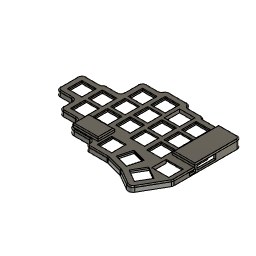
Plate (Autodesk Fusion 360 design; units mm, degrees)
Autodesk Fusion 360 part; units mm, degrees
sketch "plate-Edge_Cuts" plane through (0, 0, 0) normal (0, 0, 1) x (1, 0, 0)
  line L0 (52.0077, -29.7844) -> (52.0077, -15.8344)
  line L1 (65.9577, -29.7844) -> (52.0077, -29.7844)
  line L2 (29.9577, -38.8344) -> (29.9577, -52.7844)
  line L3 (144.4827, -45.3094) -> (142.4827, -45.3094)
  line L4 (65.9577, -49.8344) -> (65.9577, -63.7844)
  line L5 (106.0077, -65.7844) -> (106.0077, -51.8344)
  line L6 (142.4827, -45.0594) -> (144.4827, -45.0594)
  line L7 (96.4397, -85.7414) -> (100.0507, -72.2664)
  line L8 (119.9577, -48.7844) -> (106.0077, -48.7844)
  line L9 (100.0507, -72.2664) -> (113.5257, -75.8774)
  line L10 (119.9577, -34.8334) -> (119.9577, -48.7844)
  line L11 (119.9577, -51.8344) -> (119.9577, -65.7844)
  line L12 (119.9577, -65.7844) -> (106.0077, -65.7844)
  line L13 (106.0077, -34.8335) -> (119.9577, -34.8334)
  line L14 (113.5257, -75.8774) -> (109.9147, -89.3524)
  line L15 (65.9577, -63.7844) -> (52.0077, -63.7844)
  line L16 (65.9577, -15.8344) -> (65.9577, -29.7844)
  line L17 (52.0077, -49.8344) -> (65.9577, -49.8344)
  line L18 (83.9577, -25.7844) -> (70.0077, -25.7844)
  line L19 (16.0077, -52.7844) -> (16.0077, -38.8344)
  line L20 (70.0077, -25.7844) -> (70.0077, -11.8344)
  line L21 (106.0077, -48.7844) -> (106.0077, -34.8335)
  line L22 (106.0077, -51.8344) -> (119.9577, -51.8344)
  line L23 (109.9147, -89.3524) -> (96.4397, -85.7414)
  line L24 (52.0077, -63.7844) -> (52.0077, -49.8344)
  line L25 (83.9577, -11.8344) -> (83.9577, -25.7844)
  line L26 (29.9577, -52.7844) -> (16.0077, -52.7844)
  line L27 (101.9577, -63.7844) -> (88.0077, -63.7844)
  line L28 (123.4827, -78.3094) -> (123.4827, -64.3094)
  line L29 (119.9577, -17.8344) -> (119.9577, -31.7844)
  line L30 (106.0077, -31.7844) -> (106.0077, -17.8344)
  line L31 (119.9577, -31.7844) -> (106.0077, -31.7844)
  line L32 (83.9577, -28.8326) -> (83.9577, -42.7844)
  line L33 (83.9577, -59.7844) -> (70.0077, -59.7844)
  line L34 (83.9577, -42.7844) -> (70.0077, -42.7844)
  line L35 (70.0077, -42.7844) -> (70.0077, -28.8329)
  line L36 (88.0077, -49.8344) -> (101.9577, -49.8344)
  line L37 (83.9577, -45.8344) -> (83.9577, -59.7844)
  line L38 (106.0077, -17.8344) -> (119.9577, -17.8344)
  line L39 (52.0077, -15.8344) -> (65.9577, -15.8344)
  line L40 (139.9827, -78.3094) -> (123.4827, -78.3094)
  line L41 (101.9577, -49.8344) -> (101.9577, -63.7844)
  line L42 (16.0077, -38.8344) -> (29.9577, -38.8344)
  line L43 (70.0077, -11.8344) -> (83.9577, -11.8344)
  line L44 (88.0077, -63.7844) -> (88.0077, -49.8344)
  line L45 (88.0077, -15.8344) -> (101.9577, -15.8344)
  line L46 (114.4547, -91.3624) -> (121.4297, -79.2814)
  line L47 (101.9577, -32.8344) -> (101.9577, -46.7854)
  line L48 (34.0077, -36.8344) -> (47.9577, -36.8344)
  line L49 (101.9577, -46.7854) -> (88.0077, -46.7853)
  line L50 (47.9577, -53.8325) -> (47.9577, -67.7844)
  line L51 (91.4577, -71.3344) -> (91.4577, -85.2844)
  line L52 (133.5107, -86.2564) -> (126.5357, -98.3374)
  line L53 (34.0077, -53.8331) -> (47.9577, -53.8325)
  line L54 (47.9577, -67.7844) -> (34.0077, -67.7844)
  line L55 (101.9577, -15.8344) -> (101.9577, -29.7844)
  line L56 (91.4577, -85.2844) -> (77.5077, -85.2844)
  line L57 (47.9577, -36.8344) -> (47.9577, -50.7844)
  line L58 (88.0077, -29.7844) -> (88.0077, -15.8344)
  line L59 (121.4297, -79.2814) -> (133.5107, -86.2564)
  line L60 (77.5077, -71.3344) -> (91.4577, -71.3344)
  line L61 (70.0077, -45.8344) -> (83.9577, -45.8344)
  line L62 (77.5077, -85.2844) -> (77.5077, -71.3344)
  line L63 (88.0077, -46.7853) -> (88.0077, -32.8344)
  line L64 (101.9577, -29.7844) -> (88.0077, -29.7844)
  line L65 (88.0077, -32.8344) -> (101.9577, -32.8344)
  line L66 (126.5357, -98.3374) -> (114.4547, -91.3624)
  line L67 (70.0077, -59.7844) -> (70.0077, -45.8344)
  line L68 (47.9577, -50.7844) -> (34.0077, -50.7844)
  line L69 (70.0077, -28.8329) -> (83.9577, -28.8326)
  line L70 (34.0077, -67.7844) -> (34.0077, -53.8331)
  line L71 (34.0077, -50.7844) -> (34.0077, -36.8344)
  line L72 (65.9577, -46.7844) -> (52.0077, -46.7844)
  line L73 (52.0077, -46.7844) -> (52.0077, -32.8329)
  line L74 (65.9577, -32.8325) -> (65.9577, -46.7844)
  line L75 (52.0077, -32.8329) -> (65.9577, -32.8325)
  line L76 (142.4827, -57.8094) -> (144.4827, -57.8094)
  line L77 (30.4577, -38.3344) -> (30.4577, -53.2844)
  line L78 (30.4577, -53.2844) -> (15.5077, -53.2844)
  line L79 (15.5077, -53.2844) -> (15.5077, -38.3344)
  line L80 (15.5077, -38.3344) -> (30.4577, -38.3344)
  line L81 (33.5077, -36.3344) -> (48.4577, -36.3344)
  line L82 (95.8273, -86.0949) -> (99.6972, -71.654)
  line L83 (99.6972, -71.654) -> (114.1381, -75.5238)
  line L84 (114.1381, -75.5238) -> (110.2682, -89.9647)
  line L85 (110.2682, -89.9647) -> (95.8273, -86.0949)
  line L86 (105.5077, -68.2844) -> (105.5077, -51.3344)
  line L87 (105.5077, -51.3344) -> (120.4577, -51.3344)
  line L88 (120.4577, -51.3344) -> (120.4577, -68.2844)
  line L89 (120.4577, -68.2844) -> (105.5077, -68.2844)
  line L90 (105.5077, -17.3344) -> (120.4577, -17.3344)
  line L91 (87.5077, -66.2844) -> (87.5077, -32.3344)
  line L92 (87.5077, -32.3344) -> (102.4577, -32.3344)
  line L93 (102.4577, -32.3344) -> (102.4577, -66.2844)
  line L94 (69.5077, -62.7844) -> (69.5077, -45.3344)
  line L95 (69.5077, -45.3344) -> (84.4577, -45.3344)
  line L96 (84.4577, -45.3344) -> (84.4577, -62.7844)
  line L97 (84.4577, -62.7844) -> (69.5077, -62.7844)
  line L98 (69.5077, -11.3344) -> (84.4577, -11.3344)
  line L99 (66.4577, -15.3344) -> (66.4577, -47.2844)
  line L100 (66.4577, -47.2844) -> (51.5077, -47.2844)
  line L101 (51.5077, -47.2844) -> (51.5077, -15.3344)
  line L102 (48.4577, -36.3344) -> (48.4577, -68.2844)
  line L103 (48.4577, -68.2844) -> (33.5077, -68.2844)
  line L104 (33.5077, -68.2844) -> (33.5077, -36.3344)
  line L105 (66.4577, -49.3344) -> (66.4577, -64.2844)
  line L106 (66.4577, -64.2844) -> (51.5077, -64.2844)
  line L107 (51.5077, -64.2844) -> (51.5077, -49.3344)
  line L108 (51.5077, -49.3344) -> (66.4577, -49.3344)
  line L109 (51.5077, -15.3344) -> (66.4577, -15.3344)
  line L110 (69.5077, -43.2844) -> (69.5077, -11.3344)
  line L111 (84.4577, -11.3344) -> (84.4577, -43.2844)
  line L112 (84.4577, -43.2844) -> (69.5077, -43.2844)
  line L113 (102.4577, -66.2844) -> (87.5077, -66.2844)
  line L114 (87.5077, -30.2844) -> (87.5077, -15.3344)
  line L115 (87.5077, -15.3344) -> (102.4577, -15.3344)
  line L116 (102.4577, -15.3344) -> (102.4577, -30.2844)
  line L117 (102.4577, -30.2844) -> (87.5077, -30.2844)
  line L118 (105.5077, -49.2844) -> (105.5077, -17.3344)
  line L119 (120.4577, -17.3344) -> (120.4577, -49.2844)
  line L120 (120.4577, -49.2844) -> (105.5077, -49.2844)
  line L121 (77.0077, -85.7844) -> (77.0077, -68.8344)
  line L122 (77.0077, -68.8344) -> (91.9577, -68.8344)
  line L123 (91.9577, -68.8344) -> (91.9577, -85.7844)
  line L124 (91.9577, -85.7844) -> (77.0077, -85.7844)
  line L125 (113.7717, -91.5454) -> (121.2467, -78.5984)
  line L126 (121.2467, -78.5984) -> (134.1937, -86.0734)
  line L127 (134.1937, -86.0734) -> (126.7187, -99.0204)
  line L128 (126.7187, -99.0204) -> (113.7717, -91.5454)
  line L129 (51.7516, -67.7801) -> (73.7516, -67.7801)
  line L130 (73.7516, -67.7801) -> (73.7516, -80.7801)
  line L131 (73.7516, -80.7801) -> (51.7516, -80.7801)
  line L132 (51.7516, -80.7801) -> (51.7516, -67.7801)
  line L133 (75.3516, -66.1801) -> (75.3516, -82.3801)
  line L134 (75.3516, -82.3801) -> (50.1516, -82.3801)
  line L135 (50.1516, -82.3801) -> (50.1516, -66.1801)
  line L136 (50.1516, -66.1801) -> (75.3516, -66.1801)
  arc A0 (125.737, -102.2448) -> (129.1584, -101.3221) centre (126.9827, -100.0594) ccw
  arc A1 (129.1584, -101.3221) -> (129.16, -101.3193) centre (128.2935, -100.8202) ccw
  line L137 (129.16, -101.3193) -> (141.9487, -79.12)
  line L138 (142.4827, -15.8344) -> (142.4827, -77.1233)
  arc A2 (142.4827, -16.3094) -> (140.4827, -14.3094) centre (140.4827, -16.3094) ccw
  line L139 (105.4827, -14.3094) -> (140.4827, -14.3094)
  arc A3 (104.9827, -13.8094) -> (105.4827, -14.3094) centre (105.4827, -13.8094) ccw
  arc A4 (104.9827, -13.8094) -> (103.4827, -12.3094) centre (103.4827, -13.8094) ccw
  line L140 (88.4827, -12.3094) -> (103.4827, -12.3094)
  arc A5 (87.4827, -11.3094) -> (88.4827, -12.3094) centre (88.4827, -11.3094) ccw
  line L141 (87.4827, -10.3094) -> (87.4827, -11.3094)
  arc A6 (87.4827, -10.3094) -> (85.4827, -8.3094) centre (85.4827, -10.3094) ccw
  line L142 (68.4827, -8.3094) -> (85.4827, -8.3094)
  arc A7 (68.4827, -8.3094) -> (66.4827, -10.3094) centre (68.4827, -10.3094) ccw
  line L143 (66.4827, -10.3094) -> (66.4827, -11.3094)
  arc A8 (65.4827, -12.3094) -> (66.4827, -11.3094) centre (65.4827, -11.3094) ccw
  line L144 (65.4827, -12.3094) -> (50.4827, -12.3094)
  arc A9 (50.4827, -12.3094) -> (48.4827, -14.3094) centre (50.4827, -14.3094) ccw
  line L145 (48.4827, -14.3094) -> (48.4827, -32.3094)
  arc A10 (47.4827, -33.3094) -> (48.4827, -32.3094) centre (47.4827, -32.3094) ccw
  line L146 (47.4827, -33.3094) -> (32.4827, -33.3094)
  arc A11 (32.4827, -33.3094) -> (30.9827, -34.8094) centre (32.4827, -34.8094) ccw
  arc A12 (30.4827, -35.3094) -> (30.9827, -34.8094) centre (30.4827, -34.8094) ccw
  line L147 (14.4827, -35.3094) -> (30.4827, -35.3094)
  arc A13 (14.4827, -35.3094) -> (12.4827, -37.3094) centre (14.4827, -37.3094) ccw
  line L148 (12.4827, -37.3094) -> (12.4827, -54.3094)
  arc A14 (12.4827, -54.3094) -> (14.4827, -56.3094) centre (14.4827, -54.3094) ccw
  line L149 (14.4827, -56.3094) -> (29.4827, -56.3094)
  arc A15 (30.4827, -57.3094) -> (29.4827, -56.3094) centre (29.4827, -57.3094) ccw
  line L150 (30.4827, -57.3094) -> (30.4827, -69.3094)
  arc A16 (30.4827, -69.3094) -> (32.4827, -71.3094) centre (32.4827, -69.3094) ccw
  line L151 (32.4827, -71.3094) -> (50.1516, -71.3094)
  line L152 (74.9827, -88.8094) -> (92.8162, -88.8094)
  line L153 (93.995, -88.9665) -> (110.2134, -93.3687)
  line L154 (111.3021, -93.8245) -> (125.7283, -102.2398)
  arc A17 (125.7283, -102.2398) -> (125.737, -102.2448) centre (126.2322, -101.3761) ccw
  line L155 (32.4827, -73.3094) -> (44.1516, -73.3094)
  arc A18 (28.4827, -69.3094) -> (32.4827, -73.3094) centre (32.4827, -69.3094) ccw
  line L156 (28.4827, -61.3094) -> (28.4827, -69.3094)
  line L157 (14.4827, -58.3094) -> (25.4827, -58.3094)
  arc A19 (10.4827, -54.3094) -> (14.4827, -58.3094) centre (14.4827, -54.3094) ccw
  line L158 (10.4827, -37.3094) -> (10.4827, -54.3094)
  arc A20 (14.4827, -33.3094) -> (10.4827, -37.3094) centre (14.4827, -37.3094) ccw
  line L159 (14.4827, -33.3094) -> (28.7411, -33.3094)
  arc A21 (32.4827, -31.3094) -> (29.5725, -32.8649) centre (32.4827, -34.8094) ccw
  line L160 (43.4827, -31.3094) -> (32.4827, -31.3094)
  line L161 (46.4827, -14.3094) -> (46.4827, -28.3094)
  arc A22 (50.4827, -10.3094) -> (46.4827, -14.3094) centre (50.4827, -14.3094) ccw
  line L162 (62.1582, -10.3094) -> (50.4827, -10.3094)
  arc A23 (68.4827, -6.3094) -> (64.8687, -8.5951) centre (68.4827, -10.3094) ccw
  line L163 (68.4827, -6.3094) -> (85.4827, -6.3094)
  arc A24 (89.0967, -8.5951) -> (85.4827, -6.3094) centre (85.4827, -10.3094) ccw
  line L164 (91.8073, -10.3094) -> (103.4827, -10.3094)
  arc A25 (106.3929, -11.8649) -> (103.4827, -10.3094) centre (103.4827, -13.8094) ccw
  line L165 (107.2244, -12.3094) -> (140.4827, -12.3094)
  arc A26 (144.4827, -16.3094) -> (140.4827, -12.3094) centre (140.4827, -16.3094) ccw
  line L166 (144.4827, -16.3094) -> (144.4827, -77.6582)
  line L167 (130.893, -102.3177) -> (143.9487, -79.6549)
  arc A27 (130.8881, -102.3261) -> (130.893, -102.3177) centre (128.2935, -100.8202) ccw
  arc A28 (124.7466, -103.9824) -> (130.8881, -102.3261) centre (126.9827, -100.0594) ccw
  arc A29 (124.7206, -103.9674) -> (124.7466, -103.9824) centre (126.2322, -101.3761) ccw
  line L168 (110.4657, -95.6521) -> (124.7206, -103.9674)
  line L169 (93.7284, -90.9665) -> (109.498, -95.2468)
  line L170 (74.9827, -90.8094) -> (92.5496, -90.8094)
  arc A30 (48.1516, -78.3801) -> (54.1516, -84.3801) centre (54.1516, -78.3801) ccw
  line L171 (54.1516, -84.3801) -> (68.9827, -84.3801)
  line L172 (48.1516, -78.3801) -> (48.1516, -77.3094)
  arc A31 (48.1516, -77.3094) -> (44.1516, -73.3094) centre (44.1516, -77.3094) ccw
  arc A32 (71.9827, -87.3801) -> (68.9827, -84.3801) centre (68.9827, -87.3801) ccw
  arc A33 (71.9827, -87.8094) -> (74.9827, -90.8094) centre (74.9827, -87.8094) ccw
  line L173 (71.9827, -87.3801) -> (71.9827, -87.8094)
  arc A34 (106.3929, -11.8649) -> (107.2244, -12.3094) centre (107.2244, -11.3094) ccw
  arc A35 (43.4827, -31.3094) -> (46.4827, -28.3094) centre (43.4827, -28.3094) ccw
  arc A36 (28.7411, -33.3094) -> (29.5725, -32.8649) centre (28.7411, -32.3094) ccw
  line L174 (99.6972, -71.654) -> (114.1381, -75.5238)
  line L175 (77.0077, -85.7844) -> (77.0077, -68.8344)
  line L176 (101.9577, -46.7854) -> (88.0077, -46.7853)
  line L177 (95.8273, -86.0949) -> (99.6972, -71.654)
  line L178 (106.0077, -31.7844) -> (106.0077, -17.8344)
  line L179 (101.9577, -32.8344) -> (101.9577, -46.7854)
  line L180 (102.4577, -30.2844) -> (87.5077, -30.2844)
  line L181 (88.0077, -49.8344) -> (101.9577, -49.8344)
  line L182 (101.9577, -29.7844) -> (88.0077, -29.7844)
  line L183 (102.4577, -32.3344) -> (102.4577, -66.2844)
  line L184 (144.4827, -61.8094) -> (142.4827, -61.8094)
  line L185 (106.0077, -34.8335) -> (119.9577, -34.8334)
  line L186 (126.7187, -99.0204) -> (113.7717, -91.5454)
  line L187 (91.4577, -71.3344) -> (91.4577, -85.2844)
  line L188 (88.0077, -32.8344) -> (101.9577, -32.8344)
  line L189 (87.5077, -32.3344) -> (102.4577, -32.3344)
  line L190 (102.4577, -15.3344) -> (102.4577, -30.2844)
  line L191 (139.9827, -64.3094) -> (139.9827, -78.3094)
  line L192 (105.5077, -49.2844) -> (105.5077, -17.3344)
  line L193 (106.0077, -48.7844) -> (106.0077, -34.8335)
  line L194 (101.9577, -63.7844) -> (88.0077, -63.7844)
  line L195 (88.0077, -15.8344) -> (101.9577, -15.8344)
  line L196 (136.9827, -12.3094) -> (136.9827, -14.3094)
  line L197 (133.5107, -86.2564) -> (126.5357, -98.3374)
  line L198 (87.5077, -15.3344) -> (102.4577, -15.3344)
  line L199 (134.1937, -86.0734) -> (126.7187, -99.0204)
  line L200 (102.4577, -66.2844) -> (87.5077, -66.2844)
  line L201 (121.2467, -78.5984) -> (134.1937, -86.0734)
  line L202 (101.9577, -15.8344) -> (101.9577, -29.7844)
  line L203 (121.4297, -79.2814) -> (133.5107, -86.2564)
  line L204 (105.5077, -17.3344) -> (120.4577, -17.3344)
  line L205 (91.4577, -85.2844) -> (77.5077, -85.2844)
  line L206 (120.4577, -68.2844) -> (105.5077, -68.2844)
  line L207 (106.0077, -51.8344) -> (119.9577, -51.8344)
  line L208 (91.9577, -85.7844) -> (77.0077, -85.7844)
  line L209 (91.9577, -68.8344) -> (91.9577, -85.7844)
  line L210 (52.0077, -49.8344) -> (65.9577, -49.8344)
  line L211 (114.1381, -75.5238) -> (110.2682, -89.9647)
  line L212 (52.0077, -32.8329) -> (65.9577, -32.8325)
  line L213 (114.4547, -91.3624) -> (121.4297, -79.2814)
  line L214 (106.0077, -17.8344) -> (119.9577, -17.8344)
  line L215 (109.9147, -89.3524) -> (96.4397, -85.7414)
  line L216 (66.4577, -47.2844) -> (51.5077, -47.2844)
  line L217 (113.7717, -91.5454) -> (121.2467, -78.5984)
  line L218 (66.4577, -64.2844) -> (51.5077, -64.2844)
  line L219 (65.9577, -32.8325) -> (65.9577, -46.7844)
  line L220 (120.4577, -51.3344) -> (120.4577, -68.2844)
  line L221 (48.4577, -36.3344) -> (48.4577, -68.2844)
  line L222 (110.2682, -89.9647) -> (95.8273, -86.0949)
  line L223 (65.9577, -46.7844) -> (52.0077, -46.7844)
  line L224 (113.5257, -75.8774) -> (109.9147, -89.3524)
  line L225 (77.5077, -85.2844) -> (77.5077, -71.3344)
  line L226 (100.0507, -72.2664) -> (113.5257, -75.8774)
  line L227 (105.5077, -51.3344) -> (120.4577, -51.3344)
  line L228 (51.5077, -49.3344) -> (66.4577, -49.3344)
  line L229 (119.9577, -65.7844) -> (106.0077, -65.7844)
  line L230 (119.9577, -48.7844) -> (106.0077, -48.7844)
  line L231 (119.9577, -17.8344) -> (119.9577, -31.7844)
  line L232 (65.9577, -29.7844) -> (52.0077, -29.7844)
  line L233 (120.4577, -49.2844) -> (105.5077, -49.2844)
  line L234 (66.4577, -15.3344) -> (66.4577, -47.2844)
  line L235 (101.9577, -49.8344) -> (101.9577, -63.7844)
  line L236 (51.5077, -15.3344) -> (66.4577, -15.3344)
  line L237 (47.9577, -36.8344) -> (47.9577, -50.7844)
  line L238 (126.5357, -98.3374) -> (114.4547, -91.3624)
  line L239 (96.4397, -85.7414) -> (100.0507, -72.2664)
  line L240 (65.9577, -63.7844) -> (52.0077, -63.7844)
  line L241 (119.9577, -31.7844) -> (106.0077, -31.7844)
  line L242 (88.0077, -46.7853) -> (88.0077, -32.8344)
  line L243 (105.5077, -68.2844) -> (105.5077, -51.3344)
  line L244 (106.0077, -65.7844) -> (106.0077, -51.8344)
  line L245 (52.0077, -15.8344) -> (65.9577, -15.8344)
  line L246 (29.9577, -38.8344) -> (29.9577, -52.7844)
  line L247 (69.5077, -43.2844) -> (69.5077, -11.3344)
  line L248 (33.5077, -68.2844) -> (33.5077, -36.3344)
  line L249 (83.9577, -28.8326) -> (83.9577, -42.7844)
  line L250 (48.4577, -68.2844) -> (33.5077, -68.2844)
  line L251 (15.5077, -38.3344) -> (30.4577, -38.3344)
  line L252 (70.0077, -45.8344) -> (83.9577, -45.8344)
  line L253 (84.4577, -62.7844) -> (69.5077, -62.7844)
  line L254 (87.5077, -66.2844) -> (87.5077, -32.3344)
  line L255 (70.0077, -42.7844) -> (70.0077, -28.8329)
  line L256 (119.9577, -51.8344) -> (119.9577, -65.7844)
  line L257 (77.0077, -68.8344) -> (91.9577, -68.8344)
  line L258 (30.4577, -38.3344) -> (30.4577, -53.2844)
  line L259 (120.4577, -17.3344) -> (120.4577, -49.2844)
  line L260 (84.4577, -45.3344) -> (84.4577, -62.7844)
  line L261 (16.0077, -52.7844) -> (16.0077, -38.8344)
  line L262 (34.0077, -50.7844) -> (34.0077, -36.8344)
  line L263 (15.5077, -53.2844) -> (15.5077, -38.3344)
  line L264 (84.4577, -11.3344) -> (84.4577, -43.2844)
  line L265 (83.9577, -11.8344) -> (83.9577, -25.7844)
  line L266 (83.9577, -42.7844) -> (70.0077, -42.7844)
  line L267 (77.5077, -71.3344) -> (91.4577, -71.3344)
  line L268 (119.9577, -34.8334) -> (119.9577, -48.7844)
  line L269 (88.0077, -63.7844) -> (88.0077, -49.8344)
  line L270 (65.9577, -49.8344) -> (65.9577, -63.7844)
  line L271 (84.4577, -43.2844) -> (69.5077, -43.2844)
  line L272 (70.0077, -11.8344) -> (83.9577, -11.8344)
  line L273 (88.0077, -29.7844) -> (88.0077, -15.8344)
  line L274 (33.5077, -36.3344) -> (48.4577, -36.3344)
  line L275 (51.5077, -64.2844) -> (51.5077, -49.3344)
  line L276 (66.4577, -49.3344) -> (66.4577, -64.2844)
  line L277 (34.0077, -67.7844) -> (34.0077, -53.8331)
  line L278 (16.0077, -38.8344) -> (29.9577, -38.8344)
  line L279 (70.0077, -25.7844) -> (70.0077, -11.8344)
  line L280 (34.0077, -36.8344) -> (47.9577, -36.8344)
  line L281 (83.9577, -45.8344) -> (83.9577, -59.7844)
  line L282 (30.4577, -53.2844) -> (15.5077, -53.2844)
  line L283 (65.9577, -15.8344) -> (65.9577, -29.7844)
  line L284 (29.9577, -52.7844) -> (16.0077, -52.7844)
  line L285 (47.9577, -53.8325) -> (47.9577, -67.7844)
  line L286 (52.0077, -29.7844) -> (52.0077, -15.8344)
  line L287 (51.5077, -47.2844) -> (51.5077, -15.3344)
  line L288 (52.0077, -63.7844) -> (52.0077, -49.8344)
  line L289 (87.5077, -30.2844) -> (87.5077, -15.3344)
  line L290 (70.0077, -59.7844) -> (70.0077, -45.8344)
  line L291 (34.0077, -53.8331) -> (47.9577, -53.8325)
  line L292 (47.9577, -67.7844) -> (34.0077, -67.7844)
  line L293 (83.9577, -59.7844) -> (70.0077, -59.7844)
  line L294 (70.0077, -28.8329) -> (83.9577, -28.8326)
  line L295 (69.5077, -62.7844) -> (69.5077, -45.3344)
  line L296 (47.9577, -50.7844) -> (34.0077, -50.7844)
  line L297 (69.5077, -11.3344) -> (84.4577, -11.3344)
  line L298 (52.0077, -46.7844) -> (52.0077, -32.8329)
  line L299 (83.9577, -25.7844) -> (70.0077, -25.7844)
  line L300 (69.5077, -45.3344) -> (84.4577, -45.3344)
  line L301 (121.2467, -78.5984) -> (134.1937, -86.0734)
  line L302 (84.4577, -62.7844) -> (69.5077, -62.7844)
  line L303 (52.0077, -29.7844) -> (52.0077, -15.8344)
  line L304 (66.4577, -49.3344) -> (66.4577, -64.2844)
  line L305 (34.0077, -67.7844) -> (34.0077, -53.8331)
  line L306 (83.9577, -45.8344) -> (83.9577, -59.7844)
  line L307 (47.9577, -50.7844) -> (34.0077, -50.7844)
  line L308 (52.0077, -63.7844) -> (52.0077, -49.8344)
  line L309 (70.0077, -25.7844) -> (70.0077, -11.8344)
  line L310 (65.9577, -49.8344) -> (65.9577, -63.7844)
  line L311 (84.4577, -45.3344) -> (84.4577, -62.7844)
  line L312 (88.0077, -29.7844) -> (88.0077, -15.8344)
  line L313 (69.5077, -11.3344) -> (84.4577, -11.3344)
  line L314 (47.9577, -36.8344) -> (47.9577, -50.7844)
  line L315 (47.9577, -53.8325) -> (47.9577, -67.7844)
  line L316 (15.5077, -53.2844) -> (15.5077, -38.3344)
  line L317 (77.5077, -71.3344) -> (91.4577, -71.3344)
  line L318 (34.0077, -53.8331) -> (47.9577, -53.8325)
  line L319 (69.5077, -62.7844) -> (69.5077, -45.3344)
  line L320 (84.4577, -43.2844) -> (69.5077, -43.2844)
  line L321 (29.9577, -52.7844) -> (16.0077, -52.7844)
  line L322 (34.0077, -50.7844) -> (34.0077, -36.8344)
  line L323 (51.5077, -47.2844) -> (51.5077, -15.3344)
  line L324 (77.0077, -68.8344) -> (91.9577, -68.8344)
  line L325 (83.9577, -11.8344) -> (83.9577, -25.7844)
  line L326 (70.0077, -59.7844) -> (70.0077, -45.8344)
  line L327 (70.0077, -11.8344) -> (83.9577, -11.8344)
  line L328 (69.5077, -45.3344) -> (84.4577, -45.3344)
  line L329 (83.9577, -42.7844) -> (70.0077, -42.7844)
  line L330 (70.0077, -45.8344) -> (83.9577, -45.8344)
  line L331 (33.5077, -36.3344) -> (48.4577, -36.3344)
  line L332 (83.9577, -25.7844) -> (70.0077, -25.7844)
  line L333 (30.4577, -53.2844) -> (15.5077, -53.2844)
  line L334 (16.0077, -52.7844) -> (16.0077, -38.8344)
  line L335 (70.0077, -28.8329) -> (83.9577, -28.8326)
  line L336 (88.0077, -63.7844) -> (88.0077, -49.8344)
  line L337 (48.4577, -36.3344) -> (48.4577, -68.2844)
  line L338 (87.5077, -30.2844) -> (87.5077, -15.3344)
  line L339 (15.5077, -38.3344) -> (30.4577, -38.3344)
  line L340 (83.9577, -59.7844) -> (70.0077, -59.7844)
  line L341 (144.4827, -37.0594) -> (142.4827, -37.0594)
  line L342 (91.9577, -68.8344) -> (91.9577, -85.7844)
  line L343 (142.4827, -55.3094) -> (144.4827, -55.3094)
  line L344 (126.7187, -99.0204) -> (113.7717, -91.5454)
  line L345 (119.9577, -31.7844) -> (106.0077, -31.7844)
  line L346 (110.2682, -89.9647) -> (95.8273, -86.0949)
  line L347 (109.9147, -89.3524) -> (96.4397, -85.7414)
  line L348 (105.5077, -17.3344) -> (120.4577, -17.3344)
  line L349 (106.0077, -34.8335) -> (119.9577, -34.8334)
  line L350 (77.0077, -85.7844) -> (77.0077, -68.8344)
  line L351 (101.9577, -63.7844) -> (88.0077, -63.7844)
  line L352 (91.4577, -71.3344) -> (91.4577, -85.2844)
  line L353 (95.8273, -86.0949) -> (99.6972, -71.654)
  line L354 (77.5077, -85.2844) -> (77.5077, -71.3344)
  line L355 (119.9577, -65.7844) -> (106.0077, -65.7844)
  line L356 (88.0077, -32.8344) -> (101.9577, -32.8344)
  line L357 (102.4577, -30.2844) -> (87.5077, -30.2844)
  line L358 (101.9577, -46.7854) -> (88.0077, -46.7853)
  line L359 (99.6972, -71.654) -> (114.1381, -75.5238)
  line L360 (105.5077, -51.3344) -> (120.4577, -51.3344)
  line L361 (120.4577, -68.2844) -> (105.5077, -68.2844)
  line L362 (66.4577, -47.2844) -> (51.5077, -47.2844)
  line L363 (100.0507, -72.2664) -> (113.5257, -75.8774)
  line L364 (119.9577, -51.8344) -> (119.9577, -65.7844)
  line L365 (133.5107, -86.2564) -> (126.5357, -98.3374)
  line L366 (121.4297, -79.2814) -> (133.5107, -86.2564)
  line L367 (88.0077, -15.8344) -> (101.9577, -15.8344)
  line L368 (88.0077, -49.8344) -> (101.9577, -49.8344)
  line L369 (101.9577, -29.7844) -> (88.0077, -29.7844)
  line L370 (87.5077, -32.3344) -> (102.4577, -32.3344)
  line L371 (87.5077, -15.3344) -> (102.4577, -15.3344)
  line L372 (102.4577, -66.2844) -> (87.5077, -66.2844)
  line L373 (134.1937, -86.0734) -> (126.7187, -99.0204)
  line L374 (120.4577, -51.3344) -> (120.4577, -68.2844)
  line L375 (120.4577, -49.2844) -> (105.5077, -49.2844)
  line L376 (126.5357, -98.3374) -> (114.4547, -91.3624)
  line L377 (120.4577, -17.3344) -> (120.4577, -49.2844)
  line L378 (52.0077, -32.8329) -> (65.9577, -32.8325)
  line L379 (114.4547, -91.3624) -> (121.4297, -79.2814)
  line L380 (65.9577, -46.7844) -> (52.0077, -46.7844)
  line L381 (66.4577, -64.2844) -> (51.5077, -64.2844)
  line L382 (51.5077, -49.3344) -> (66.4577, -49.3344)
  line L383 (52.0077, -15.8344) -> (65.9577, -15.8344)
  line L384 (70.0077, -42.7844) -> (70.0077, -28.8329)
  line L385 (66.4577, -15.3344) -> (66.4577, -47.2844)
  line L386 (52.0077, -49.8344) -> (65.9577, -49.8344)
  line L387 (101.9577, -49.8344) -> (101.9577, -63.7844)
  line L388 (91.4577, -85.2844) -> (77.5077, -85.2844)
  line L389 (105.5077, -49.2844) -> (105.5077, -17.3344)
  line L390 (106.0077, -31.7844) -> (106.0077, -17.8344)
  line L391 (51.5077, -15.3344) -> (66.4577, -15.3344)
  line L392 (101.9577, -32.8344) -> (101.9577, -46.7854)
  line L393 (113.7717, -91.5454) -> (121.2467, -78.5984)
  line L394 (114.1381, -75.5238) -> (110.2682, -89.9647)
  line L395 (91.9577, -85.7844) -> (77.0077, -85.7844)
  line L396 (65.9577, -29.7844) -> (52.0077, -29.7844)
  line L397 (106.0077, -65.7844) -> (106.0077, -51.8344)
  line L398 (106.0077, -51.8344) -> (119.9577, -51.8344)
  line L399 (102.4577, -15.3344) -> (102.4577, -30.2844)
  line L400 (30.4577, -38.3344) -> (30.4577, -53.2844)
  line L401 (84.4577, -11.3344) -> (84.4577, -43.2844)
  line L402 (29.9577, -38.8344) -> (29.9577, -52.7844)
  line L403 (106.0077, -48.7844) -> (106.0077, -34.8335)
  line L404 (96.4397, -85.7414) -> (100.0507, -72.2664)
  line L405 (113.5257, -75.8774) -> (109.9147, -89.3524)
  line L406 (65.9577, -63.7844) -> (52.0077, -63.7844)
  line L407 (83.9577, -28.8326) -> (83.9577, -42.7844)
  line L408 (33.5077, -68.2844) -> (33.5077, -36.3344)
  line L409 (65.9577, -15.8344) -> (65.9577, -29.7844)
  line L410 (69.5077, -43.2844) -> (69.5077, -11.3344)
  line L411 (88.0077, -46.7853) -> (88.0077, -32.8344)
  line L412 (101.9577, -15.8344) -> (101.9577, -29.7844)
  line L413 (102.4577, -32.3344) -> (102.4577, -66.2844)
  line L414 (119.9577, -34.8334) -> (119.9577, -48.7844)
  line L415 (119.9577, -17.8344) -> (119.9577, -31.7844)
  line L416 (87.5077, -66.2844) -> (87.5077, -32.3344)
  line L417 (65.9577, -32.8325) -> (65.9577, -46.7844)
  line L418 (106.0077, -17.8344) -> (119.9577, -17.8344)
  line L419 (105.5077, -68.2844) -> (105.5077, -51.3344)
  line L420 (119.9577, -48.7844) -> (106.0077, -48.7844)
  line L421 (51.5077, -64.2844) -> (51.5077, -49.3344)
  line L422 (47.9577, -67.7844) -> (34.0077, -67.7844)
  line L423 (34.0077, -36.8344) -> (47.9577, -36.8344)
  line L424 (48.4577, -68.2844) -> (33.5077, -68.2844)
  line L425 (16.0077, -38.8344) -> (29.9577, -38.8344)
  line L426 (52.0077, -46.7844) -> (52.0077, -32.8329)
  arc A37 (50.1516, -77.3094) -> (44.1516, -71.3094) centre (44.1516, -77.3094) ccw
  line L427 (50.1516, -78.3801) -> (50.1516, -77.3094)
  arc A38 (50.1516, -78.3801) -> (54.1516, -82.3801) centre (54.1516, -78.3801) ccw
  line L428 (54.1516, -82.3801) -> (68.9827, -82.3801)
  arc A39 (73.9827, -87.3801) -> (68.9827, -82.3801) centre (68.9827, -87.3801) ccw
  line L429 (73.9827, -87.3801) -> (73.9827, -87.8094)
  arc A40 (73.9827, -87.8094) -> (74.9827, -88.8094) centre (74.9827, -87.8094) ccw
  line L430 (122.4947, -12.3094) -> (122.4947, -64.3094)
  line L431 (126.9827, -14.3094) -> (126.9827, -12.3094)
  line L432 (123.9947, -47.999) -> (132.0158, -47.999)
  line L433 (132.0158, -47.999) -> (132.0158, -55.999)
  line L434 (144.4827, -55.999) -> (123.9947, -55.999)
  line L435 (123.9947, -12.3094) -> (123.9947, -55.999)
  line L436 (144.4827, -57.499) -> (122.4947, -57.499)
  line L437 (122.4947, -64.3094) -> (142.4827, -64.3094)
  arc A41 (141.9487, -79.12) -> (142.4827, -77.1233) centre (138.4827, -77.1233) ccw
  arc A42 (143.9487, -79.6549) -> (144.4827, -77.6582) centre (140.4827, -77.6582) ccw
  arc A43 (93.7284, -90.9665) -> (92.5496, -90.8094) centre (92.5496, -95.3094) ccw
  arc A44 (110.4657, -95.6521) -> (109.498, -95.2468) centre (108.4502, -99.1072) ccw
  arc A45 (93.995, -88.9665) -> (92.8162, -88.8094) centre (92.8162, -93.3094) ccw
  arc A46 (111.3021, -93.8245) -> (110.2134, -93.3687) centre (109.0347, -97.7115) ccw
  arc A47 (28.4827, -61.3094) -> (25.4827, -58.3094) centre (25.4827, -61.3094) ccw
  arc A48 (62.1582, -10.3094) -> (64.8687, -8.5951) centre (62.1582, -7.3094) ccw
  arc A49 (89.0967, -8.5951) -> (91.8073, -10.3094) centre (91.8073, -7.3094) ccw
  dimension "d5" = 22
  dimension "d6" = 13
  dimension "d12" = 4
  dimension "d13" = 3
  dimension "d14" = 3
  dimension "d16" = 1
  dimension "d17" = 3
  dimension "d18" = 1
  dimension "d19" = 0.5
  dimension "d20" = 0.5
  dimension "d21" = 0.5
  dimension "d22" = 0.5
  dimension "d23" = 0.5
  dimension "d24" = 0.5
  dimension "d25" = 0.5
  dimension "d26" = 0.5
  dimension "d27" = 0.5
  dimension "d28" = 0.5
  dimension "d29" = 0.5
  dimension "d30" = 0.5
  dimension "d31" = 0.5
  dimension "d32" = 0.5
  dimension "d33" = 0.5
  dimension "d34" = 0.5
  dimension "d35" = 0.5
  dimension "d36" = 0.5
  dimension "d37" = 0.5
  dimension "d38" = 0.5
  dimension "d39" = 0.5
  dimension "d40" = 0.5
  dimension "d41" = 0.5
  dimension "d42" = 0.5
  dimension "d43" = 0.5
  dimension "d44" = 0.5
  dimension "d45" = 0.5
  dimension "d46" = 0.5
  dimension "d47" = 0.5
  dimension "d48" = 0.5
  dimension "d49" = 0.5
  dimension "d50" = 0.5
  dimension "d51" = 0.5
  dimension "d52" = 0.5
  dimension "d53" = 0.5
  dimension "d54" = 0.5
  dimension "d55" = 0.5
  dimension "d56" = 0.5
  dimension "d57" = 0.5
  dimension "d58" = 0.5
  dimension "d59" = 0.5
  dimension "d60" = 0.5
  dimension "d61" = 0.5
  dimension "d62" = 0.5
  dimension "d63" = 0.5
  dimension "d64" = 0.5
  dimension "d65" = 0.5
  dimension "d66" = 0.5
  dimension "d67" = 0.5
  dimension "d68" = 0.5
  dimension "d69" = 0.5
  dimension "d70" = 0.5
  dimension "d71" = 0.5
  dimension "d72" = 0.5
  dimension "d73" = 0.5
  dimension "d74" = 0.5
  dimension "d75" = 0.5
  dimension "d76" = 0.5
  dimension "d77" = 0.5
  dimension "d78" = 0.5
  dimension "d79" = 0.5
  dimension "d80" = 0.5
  dimension "d81" = 0.5
  dimension "d82" = 0.5
  dimension "d83" = 0.5
  dimension "d84" = 0.5
  dimension "d85" = 0.5
  dimension "d86" = 0.5
  dimension "d87" = 0.5
  dimension "d88" = 0.5
  dimension "d89" = 0.5
  dimension "d90" = 0.5
  dimension "d91" = 0.5
  dimension "d92" = 0.5
  dimension "d93" = 0.5
  dimension "d94" = 0.5
  dimension "d95" = 0.5
  dimension "d96" = 0.5
  dimension "d97" = 0.5
  dimension "d98" = 0.5
  dimension "d99" = 0.5
  dimension "d100" = 0.5
  dimension "d101" = 0.5
  dimension "d102" = 0.5
  dimension "d103" = 0.5
  dimension "d104" = 0.5
  dimension "d105" = 0.5
  dimension "d106" = 0.5
  dimension "d107" = 0.5
  dimension "d108" = 0.5
  dimension "d109" = 0.5
  dimension "d110" = 0.5
  dimension "d111" = 0.5
  dimension "d112" = 0.5
  dimension "d113" = 0.5
  dimension "d114" = 0.5
  dimension "d115" = -2
  dimension "d172" = 4
  dimension "d173" = 4
  dimension "d174" = 4.5
  dimension "d175" = 4
  dimension "d176" = 4.5
  dimension "d177" = 4.5
  dimension "d178" = 3
  dimension "d179" = 3
  dimension "d180" = 3
  constraint horizontal L129
  constraint vertical L130
  constraint horizontal L131
  constraint vertical L132
  constraint tangent L139 A3
  constraint tangent A4 L140
  constraint tangent A6 L142
  constraint tangent A3 A4
  constraint tangent L138 A2
  constraint tangent A2 L139
  constraint tangent A8 L144
  constraint tangent L140 A5
  constraint tangent A7 L143
  constraint tangent A5 L141
  constraint tangent L141 A6
  constraint tangent L142 A7
  constraint tangent L146 A11
  constraint tangent L143 A8
  constraint tangent L147 A13
  constraint tangent L144 A9
  constraint tangent A9 L145
  constraint tangent L145 A10
  constraint tangent A10 L146
  constraint tangent A11 A12
  constraint tangent A12 L147
  constraint tangent A13 L148
  constraint tangent L148 A14
  constraint tangent A14 L149
  constraint tangent A16 L151
  constraint tangent L149 A15
  constraint tangent A15 L150
  constraint tangent L150 A16
  constraint tangent A30 L171
  constraint tangent A30 L172
  constraint perpendicular L155 L172
  constraint concentric A16 A18
  constraint concentric A14 A19
  constraint concentric A13 A20
  constraint concentric A11 A21
  constraint concentric A9 A22
  constraint concentric A7 A23
  constraint concentric A6 A24
  constraint concentric A4 A25
  constraint concentric A2 A26
  constraint concentric A1 A27
  constraint concentric A0 A28
  constraint concentric A17 A29
  constraint tangent L157 A19
  constraint tangent A18 L156
  constraint tangent A19 L158
  constraint tangent L155 A18
  constraint tangent A21 L160
  constraint tangent L158 A20
  constraint tangent A20 L159
  constraint tangent L161 A22
  constraint tangent A22 L162
  constraint tangent A23 L163
  constraint tangent L163 A24
  constraint tangent L165 A26
  constraint tangent A26 L166
  constraint tangent L155 A31
  constraint tangent L172 A31
  constraint tangent L171 A32
  constraint tangent L170 A33
  constraint tangent A33 L173
  constraint coincident L135 L151.end
  constraint tangent L165 A34
  constraint tangent A25 A34
  constraint tangent L160 A35
  constraint tangent L161 A35
  constraint tangent L159 A36
  constraint tangent A21 A36
  constraint coincident L166 L184.start
  constraint coincident L166 L76.end
  constraint coincident L166 L341.start
  constraint coincident A2.start L138
  constraint coincident L166 L6.end
  constraint coincident L166 L3.start
  constraint coincident L166 L343.end
  constraint coincident L165 L430.start
  constraint perpendicular L165 L430
  constraint coincident L139 L431.start
  constraint coincident L139 L196.end
  constraint coincident L138 L341.end
  constraint coincident L138 L6.start
  constraint horizontal L432
  constraint vertical L433
  constraint horizontal L434
  constraint coincident L138 L184.end
  constraint coincident L138 L76.start
  constraint coincident L138 L3.end
  constraint coincident L138 L343.start
  constraint coincident L435 L432.start
  constraint coincident L433.end L434
  constraint coincident L166 L434.start
  constraint coincident L430 L436.end
  constraint coincident L28.end L437
  constraint coincident L138 L437.end
  constraint coincident L191.start L437
  constraint tangent L138 A41
  constraint tangent L137 A41
  constraint tangent L166 A42
  constraint tangent L167 A42
  constraint tangent L170 A43
  constraint tangent L169 A43
  constraint tangent L169 A44
  constraint tangent L168 A44
  constraint tangent L152 A45
  constraint tangent L153 A45
  constraint tangent L153 A46
  constraint tangent L154 A46
  constraint tangent L157 A47
  constraint tangent L156 A47
  constraint tangent L162 A48
  constraint tangent A23 A48
  constraint tangent L164 A49
  constraint tangent A24 A49
  measures "d5" distance of L129.start L129.end
  measures "d6" distance of L129.start L131.end
  measures "d12" radius of A31
  measures "d13" radius of A32
  measures "d14" radius of A33
  measures "d16" radius of A34
  measures "d17" radius of A35
  measures "d18" radius of A36
  measures "d19" distance of L246 L258
  measures "d20" distance of L282 L284
  measures "d21" distance of L261 L263
  measures "d22" distance of L251 L278
  measures "d23" distance of L274 L280
  measures "d24" distance of L177 L239
  measures "d25" distance of L174 L226
  measures "d26" distance of L211 L224
  measures "d27" distance of L215 L222
  measures "d28" distance of L243 L244
  measures "d29" distance of L207 L227
  measures "d30" distance of L220 L256
  measures "d31" distance of L204 L214
  measures "d32" distance of L242 L254
  measures "d33" distance of L188 L189
  measures "d34" distance of L179 L183
  measures "d35" distance of L290 L295
  measures "d36" distance of L252 L300
  measures "d37" distance of L260 L281
  measures "d38" distance of L272 L297
  measures "d39" distance of L219 L234
  measures "d40" distance of L216 L223
  measures "d41" distance of L287 L298
  measures "d42" distance of L221 L285
  measures "d43" distance of L250 L292
  measures "d44" distance of L248 L277
  measures "d45" distance of L270 L276
  measures "d46" distance of L218 L240
  measures "d47" distance of L275 L288
  measures "d48" distance of L210 L228
  measures "d49" distance of L236 L245
  measures "d50" distance of L247 L255
  measures "d51" distance of L249 L264
  measures "d52" distance of L266 L271
  measures "d53" distance of L273 L289
  measures "d54" distance of L195 L198
  measures "d55" distance of L190 L202
  measures "d56" distance of L180 L182
  measures "d57" distance of L192 L193
  measures "d58" distance of L259 L268
  measures "d59" distance of L230 L233
  measures "d60" distance of L175 L225
  measures "d61" distance of L187 L209
  measures "d62" distance of L205 L208
  measures "d63" distance of L213 L217
  measures "d64" distance of L201 L203
  measures "d65" distance of L197 L199
  measures "d66" distance of L186 L238
  measures "d67" distance of L400 L402
  measures "d68" distance of L321 L333
  measures "d69" distance of L316 L334
  measures "d70" distance of L339 L425
  measures "d71" distance of L331 L423
  measures "d72" distance of L353 L404
  measures "d73" distance of L359 L363
  measures "d74" distance of L394 L405
  measures "d75" distance of L346 L347
  measures "d76" distance of L397 L419
  measures "d77" distance of L360 L398
  measures "d78" distance of L364 L374
  measures "d79" distance of L348 L418
  measures "d80" distance of L411 L416
  measures "d81" distance of L356 L370
  measures "d82" distance of L392 L413
  measures "d83" distance of L319 L326
  measures "d84" distance of L328 L330
  measures "d85" distance of L306 L311
  measures "d86" distance of L313 L327
  measures "d87" distance of L385 L417
  measures "d88" distance of L362 L380
  measures "d89" distance of L323 L426
  measures "d90" distance of L315 L337
  measures "d91" distance of L422 L424
  measures "d92" distance of L305 L408
  measures "d93" distance of L304 L310
  measures "d94" distance of L381 L406
  measures "d95" distance of L308 L421
  measures "d96" distance of L382 L386
  measures "d97" distance of L383 L391
  measures "d98" distance of L384 L410
  measures "d99" distance of L401 L407
  measures "d100" distance of L320 L329
  measures "d101" distance of L312 L338
  measures "d102" distance of L367 L371
  measures "d103" distance of L399 L412
  measures "d104" distance of L357 L369
  measures "d105" distance of L389 L403
  measures "d106" distance of L377 L414
  measures "d107" distance of L375 L420
  measures "d108" distance of L350 L354
  measures "d109" distance of L342 L352
  measures "d110" distance of L388 L395
  measures "d111" distance of L379 L393
  measures "d112" distance of L301 L366
  measures "d113" distance of L365 L373
  measures "d114" distance of L344 L376
  measures "d172" radius of A41
  measures "d173" radius of A42
  measures "d174" radius of A43
  measures "d175" radius of A44
  measures "d176" radius of A45
  measures "d177" radius of A46
  measures "d178" radius of A47
  measures "d179" radius of A48
  measures "d180" radius of A49
extrude "Extrude1" add sketch "plate-Edge_Cuts" against normal blind 3.25 contours L28 L40 L133 L134 L135 L136 A0 A1 L137 L138 L139 A3 A4 L140 A5 L141 A6 L142 A7 L143 A8 L144 A9 L145 A10 L146 A11 A12 L147 A13 L148 A14 L149 A15 L150 A16 L151 L152 L153 L154 A17 L191 A39 L429 A40 L430 L437 A41 A45 A46 | L135 L151 A37
extrude "Extrude2" add sketch "plate-Edge_Cuts" against normal blind 1.25 contours L138 L139 L430 L434 L435 L436 | L138 L430 L436 L437 | L133 L134 L135 L136 L427 A38 L428 | L134 L135 A38 | L77 L78 L79 L80 L251 L258 L263 L282 L316 L333 L339 L400 | L81 L102 L103 L104 L221 L248 L250 L274 L331 L337 L408 L424 | L82 L83 L84 L85 L174 L177 L211 L222 L346 L353 L359 L394 | L86 L87 L88 L89 L206 L220 L227 L243 L360 L361 L374 L419 | L90 L118 L119 L120 L192 L204 L233 L259 L348 L375 L377 L389 | L91 L92 L93 L113 L183 L189 L200 L254 L370 L372 L413 L416 | L94 L95 L96 L97 L253 L260 L295 L300 L302 L311 L319 L328 | L98 L110 L111 L112 L247 L264 L271 L297 L313 L320 L401 L410 | L99 L100 L101 L109 L216 L234 L236 L287 L323 L362 L385 L391 | L105 L106 L107 L108 L218 L228 L275 L276 L304 L381 L382 L421 | L121 L122 L123 L124 L175 L208 L209 L257 L324 L342 L350 L395 | L125 L126 L127 L128 L186 L199 L201 L217 L301 L344 L373 L393
extrude "Extrude4" add sketch "plate-Edge_Cuts" against normal blind 3.25 contours L133 L134 L135 L136 L427 A38 L428 | L134 L135 A38
extrude "Extrude5" add sketch "plate-Edge_Cuts" along normal blind 3 contours L133 L134 L135 L136 L427 A38 L428 | L134 L135 A38 | L129 L130 L131 L132
extrude "Extrude6" cut sketch "plate-Edge_Cuts" along normal blind 1.5 contours L129 L130 L131 L132
extrude "Extrude7" add sketch "plate-Edge_Cuts" along normal blind 3 contours L138 L139 L430 L434 L435 L436 | L138 L430 L436 L437
extrude "Extrude8" add sketch "plate-Edge_Cuts" along normal blind 1.5 from surface at 1.5 contours L138 A2 L139 L432 L433 L434 L435 | L432 L433 L434 L435
extrude "Extrude9" add sketch "plate-Edge_Cuts" against normal blind 5 contours L3 L138 L166 L343 | L6 L138 L166 L341 | L138 L166 L343 L434 | L138 A2 L139 L165 A26 L166 L196 L341 | L138 L166 L434 L436 | L76 L138 L166 L436 | L76 L138 L166 L184 | L139 L165 L196 L431 | L134 L135 A0 A1 L137 L138 L139 A3 A4 L140 A5 L141 A6 L142 A7 L143 A8 L144 A9 L145 A10 L146 A11 A12 L147 A13 L148 A14 L149 A15 L150 A16 L151 L152 L153 L154 A17 L155 A18 L156 L157 A19 L158 A20 L159 A21 L160 L161 A22 L162 A23 L163 A24 L164 A25 L165 L166 L167 A27 A28 A29 L168 L169 L170 A30 L171 L172 A31 A32 A33 L173 A34 A35 A36 L184 A37 L427 L428 A39 L429 A40 L430 A41 A42 A43 A44 A45 A46 A47 A48 A49 | L139 L165 L430 L435 | L139 L165 L431 L435
extrude "Extrude10" add sketch "plate-Edge_Cuts" along normal blind 3 contours L3 L138 L166 L343 | L6 L138 L166 L341 | L138 L166 L343 L434 | L138 A2 L139 L165 A26 L166 L196 L341 | L138 L166 L434 L436 | L76 L138 L166 L436 | L76 L138 L166 L184 | L139 L165 L196 L431 | L134 L135 A0 A1 L137 L138 L139 A3 A4 L140 A5 L141 A6 L142 A7 L143 A8 L144 A9 L145 A10 L146 A11 A12 L147 A13 L148 A14 L149 A15 L150 A16 L151 L152 L153 L154 A17 L155 A18 L156 L157 A19 L158 A20 L159 A21 L160 L161 A22 L162 A23 L163 A24 L164 A25 L165 L166 L167 A27 A28 A29 L168 L169 L170 A30 L171 L172 A31 A32 A33 L173 A34 A35 A36 L184 A37 L427 L428 A39 L429 A40 L430 A41 A42 A43 A44 A45 A46 A47 A48 A49 | L139 L165 L430 L435 | L139 L165 L431 L435
extrude "Extrude11" add sketch "plate-Edge_Cuts" along normal blind 3 contours L3 L6 L138 L166
extrude "Extrude12" add sketch "plate-Edge_Cuts" against normal blind 5 contours L3 L6 L138 L166
extrude "Extrude13" add sketch "plate-Edge_Cuts" along normal blind 3 contours L432 L433 L434 L435
extrude "Extrude14" add sketch "plate-Edge_Cuts" against normal blind 3.25 contours L432 L433 L434 L435
extrude "Extrude15" cut sketch "plate-Edge_Cuts" along normal blind 3 contours L0 L1 L16 L39 L232 L245 L283 L286 L303 L383 L396 L409 | L2 L19 L26 L42 L246 L261 L278 L284 L321 L334 L402 L425 | L3 L138 L166 L343 | L3 L6 L138 L166 | L138 A2 L139 L432 L433 L434 L435 | L6 L138 L166 L341 | L138 L166 L343 L434 | L138 A2 L139 L165 A26 L166 L196 L341 | L138 L166 L434 L436 | L138 L139 L430 L434 L435 L436 | L76 L138 L166 L436 | L138 L430 L436 L437 | L432 L433 L434 L435 | L76 L138 L166 L184 | L28 L40 L133 L134 L135 L136 A0 A1 L137 L138 L139 A3 A4 L140 A5 L141 A6 L142 A7 L143 A8 L144 A9 L145 A10 L146 A11 A12 L147 A13 L148 A14 L149 A15 L150 A16 L151 L152 L153 L154 A17 L191 A39 L429 A40 L430 L437 A41 A45 A46 | L139 L165 L196 L431 | L134 L135 A0 A1 L137 L138 L139 A3 A4 L140 A5 L141 A6 L142 A7 L143 A8 L144 A9 L145 A10 L146 A11 A12 L147 A13 L148 A14 L149 A15 L150 A16 L151 L152 L153 L154 A17 L155 A18 L156 L157 A19 L158 A20 L159 A21 L160 L161 A22 L162 A23 L163 A24 L164 A25 L165 L166 L167 A27 A28 A29 L168 L169 L170 A30 L171 L172 A31 A32 A33 L173 A34 A35 A36 L184 A37 L427 L428 A39 L429 A40 L430 A41 A42 A43 A44 A45 A46 A47 A48 A49 | L139 L165 L430 L435 | L139 L165 L431 L435 | L28 L40 L191 L437 | L133 L134 L135 L136 L427 A38 L428 | L134 L135 A38 | L4 L15 L17 L24 L210 L240 L270 L288 L308 L310 L386 L406 | L5 L11 L12 L22 L207 L229 L244 L256 L355 L364 L397 L398 | L7 L9 L14 L23 L215 L224 L226 L239 L347 L363 L404 L405 | L8 L10 L13 L21 L185 L193 L230 L268 L349 L403 L414 L420 | L18 L20 L25 L43 L265 L272 L279 L299 L309 L325 L327 L332 | L27 L36 L41 L44 L181 L194 L235 L269 L336 L351 L368 L387 | L29 L30 L31 L38 L178 L214 L231 L241 L345 L390 L415 L418 | L32 L34 L35 L69 L249 L255 L266 L294 L329 L335 L384 L407 | L33 L37 L61 L67 L252 L281 L290 L293 L306 L326 L330 L340 | L45 L55 L58 L64 L182 L195 L202 L273 L312 L367 L369 L412 | L46 L52 L59 L66 L197 L203 L213 L238 L365 L366 L376 L379 | L47 L49 L63 L65 L176 L179 L188 L242 L356 L358 L392 L411 | L48 L57 L68 L71 L237 L262 L280 L296 L307 L314 L322 L423 | L50 L53 L54 L70 L277 L285 L291 L292 L305 L315 L318 L422 | L51 L56 L60 L62 L187 L205 L225 L267 L317 L352 L354 L388 | L72 L73 L74 L75 L212 L219 L223 L298 L378 L380 L417 L426 | L77 L78 L79 L80 L251 L258 L263 L282 L316 L333 L339 L400 | L81 L102 L103 L104 L221 L248 L250 L274 L331 L337 L408 L424 | L82 L83 L84 L85 L174 L177 L211 L222 L346 L353 L359 L394 | L86 L87 L88 L89 L206 L220 L227 L243 L360 L361 L374 L419 | L90 L118 L119 L120 L192 L204 L233 L259 L348 L375 L377 L389 | L91 L92 L93 L113 L183 L189 L200 L254 L370 L372 L413 L416 | L94 L95 L96 L97 L253 L260 L295 L300 L302 L311 L319 L328 | L98 L110 L111 L112 L247 L264 L271 L297 L313 L320 L401 L410 | L99 L100 L101 L109 L216 L234 L236 L287 L323 L362 L385 L391 | L105 L106 L107 L108 L218 L228 L275 L276 L304 L381 L382 L421 | L114 L115 L116 L117 L180 L190 L198 L289 L338 L357 L371 L399 | L121 L122 L123 L124 L175 L208 L209 L257 L324 L342 L350 L395 | L125 L126 L127 L128 L186 L199 L201 L217 L301 L344 L373 L393 | L129 L130 L131 L132
extrude "Extrude16" add sketch "plate-Edge_Cuts" along normal blind 3 contours L3 L138 L166 L343 | L3 L6 L138 L166 | L6 L138 L166 L341 | L138 L166 L343 L434 | L138 A2 L139 L165 A26 L166 L196 L341 | L138 L166 L434 L436 | L139 L165 L196 L431 | L139 L165 L430 L435 | L139 L165 L431 L435
extrude "Extrude17" cut sketch "plate-Edge_Cuts" along normal blind 3 contours L138 L430 L436 L437
extrude "Extrude18" cut sketch "plate-Edge_Cuts" along normal blind 5 from surface at -3.25 contours L139 L165 L196 L431
extrude "Extrude19" cut sketch "plate-Edge_Cuts" along normal blind 5 from surface at -3.25 contours L6 L138 L166 L341
extrude "Extrude20" cut sketch "plate-Edge_Cuts" along normal blind 4 from surface at -3.25 contours L3 L138 L166 L343
extrude "Extrude21" cut sketch "plate-Edge_Cuts" along normal blind 4 from surface at -3.25 contours L3 L6 L138 L166
extrude "Extrude22" cut sketch "plate-Edge_Cuts" along normal blind 2 from surface at -3.25 contours L76 L138 L166 L184
fillet "Fillet1" radius 1 5 edges at (122.4947, -13.3094, 3) (143.4827, -57.499, 3) (144.4827, -36.9042, 3) (143.3111, -13.4809, 3) (131.4887, -12.3094, 3)
extrude "Extrude23" add sketch "plate-Edge_Cuts" along normal blind 3 contours L138 A2 L139 L432 L433 L434 L435 | L138 L139 L430 L434 L435 L436 | L432 L433 L434 L435
extrude "Extrude24" cut sketch "plate-Edge_Cuts" along normal blind 1.5 contours L138 A2 L139 L432 L433 L434 L435
fillet "Fillet2" radius 1 2 edges at (132.4887, -57.499, 3) (122.4947, -35.9042, 3)
fillet "Fillet3" radius 1 43 edges at (144.4827, -67.5786, 0) (144.3469, -78.6917, 0) (137.4208, -90.9863, 0) (130.8906, -102.3219, 0) (128.1585, -104.4192, 0) (124.7336, -103.9749, 0) (117.5932, -99.8097, 0) (109.9952, -95.4176, 0) (101.6132, -93.1067, 0) (93.1442, -90.8488, 0) (83.7662, -90.8094, 0) (72.8614, -89.9307, 0) (71.9827, -87.5947, 0) (71.104, -85.2588, 0) (61.5672, -84.3801, 0) (49.9089, -82.6227, 0) (48.1516, -77.8447, 0) (46.98, -74.4809, 0) (38.3172, -73.3094, 0) (29.6543, -72.1378, 0) (28.4827, -65.3094, 0) (27.604, -59.188, 0) (19.9827, -58.3094, 0) (11.6543, -57.1378, 0) (10.4827, -45.8094, 0) (11.6543, -34.4809, 0) (21.6119, -33.3094, 0) (29.2125, -33.1913, 0) (30.8328, -31.7227, 0) (37.9827, -31.3094, 0) (45.604, -30.4307, 0) (46.4827, -21.3094, 0) (47.6543, -11.4809, 0) (56.3204, -10.3094, 0) (63.7617, -9.8448, 0) (66.3446, -6.9288, 0) (76.9827, -6.3094, 0) (87.6208, -6.9288, 0) (90.2037, -9.8448, 0) (97.645, -10.3094, 0) (105.1326, -10.7227, 0) (106.753, -12.1913, 0) (114.8596, -12.3094, 0)
extrude "Extrude25" add sketch "plate-Edge_Cuts" along normal blind 3 contours L133 L134 L135 L136 L427 A38 L428 | L134 L135 A38 | L129 L130 L131 L132
extrude "Extrude26" cut sketch "plate-Edge_Cuts" along normal blind 1.5 contours L129 L130 L131 L132
fillet "Fillet4" radius 1 5 edges at (62.7516, -82.3801, 3) (50.1516, -74.2801, 3) (50.1516, -82.3801, 1.5) (62.7516, -66.1801, 3) (75.3516, -74.2801, 3)
extrude "Extrude27" add sketch "plate-Edge_Cuts" against normal blind 5 contours L134 L135 A38
chamfer "Chamfer1" distance 1 angle 45 3 edges at (144.4827, -59.8094, -3.25) (144.4827, -61.8094, -2.25) (144.4827, -57.8094, -2.25)
fillet "Fillet5" radius 1 2 edges at (143.4827, -55.3094, -3.25) (143.4827, -55.3094, 0.75)
fillet "Fillet6" radius 1 4 edges at (136.9827, -13.3094, -3.25) (136.9827, -13.3094, 1.75) (126.9827, -13.3094, 1.75) (126.9827, -13.3094, -3.25)
